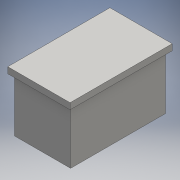
# Autodesk Inventor part: P8341 IEC with integrated fuse and switch
Saved by Autodesk Inventor 2016 (Build 200138000, 138)
## iProperties
Created: 2016-04-18
Part Number: P8341 IEC with integrated fuse and switch
Material: Generic
Document SubType Name: Modeling
Designer: Jarrett
Density: 1 g/cm^3
Appearance: Default
Author: Jarrett
Autodesk Inventor part; units mm, degrees
ref_plane "YZ Plane" through (0, 0, 0) normal (1, 0, 0) x (0, 1, 0)
ref_plane "XZ Plane" through (0, 0, 0) normal (0, 1, 0) x (-1, 0, 0)
ref_plane "XY Plane" through (0, 0, 0) normal (0, 0, 1) x (1, 0, 0)
sketch "Sketch1" plane through (0, 0, 0) normal (0, 0, 1) x (1, 0, 0)
  line L0 (0, 0) -> (30.5, 0)
  line L1 (30.5, 0) -> (30.5, 50)
  line L2 (30.5, 50) -> (0, 50)
  line L3 (0, 50) -> (0, 0)
  dimension "d0" = 50
  dimension "d1" = 30.5
  constraints: 8 end point, 2 parallel, 1 horizontal, 1 perpendicular
  measures "d0" distance of L2.end L0.start
  measures "d1" distance of L1.end L2.end
extrude "Extrusion1" add sketch "Sketch1" against normal blind 3
sketch "Sketch2" plane through (0, 0, -3) normal (0, 0, -1) x (-1, 0, 0)
  line L0 (-30.5, 50) -> (-30.5, 0) projected
  line L1 (-30.5, 25) -> (0, 25) construction
  line L2 (0, 0) -> (0, 50) projected
  line L3 (0, 50) -> (-30.5, 50) projected
  line L4 (-15.25, 50) -> (-15.25, 0) construction
  line L5 (-30.5, 0) -> (0, 0) projected
  line L6 (-28.95, 1.8) -> (-1.55, 1.8)
  line L7 (-1.55, 1.8) -> (-1.55, 48.2)
  line L8 (-1.55, 48.2) -> (-28.95, 48.2)
  line L9 (-28.95, 48.2) -> (-28.95, 1.8)
  line L10 (-28.95, 1.8) -> (-1.55, 48.2) construction
  line L11 (-1.55, 1.8) -> (-28.95, 48.2) construction
  point P0 (-15.25, 25)
  dimension "d4" = 27.4
  dimension "d5" = 46.4
  constraints: 16 end point, 7 midpoint, 2 parallel, 1 horizontal, 1 perpendicular
  measures "d4" distance of L7.end L8.end
  measures "d5" distance of L6.end L7.end
extrude "Extrusion2" add sketch "Sketch2" along normal blind 26.5 contours L9 L8 L7 L6
body "Solid1"
